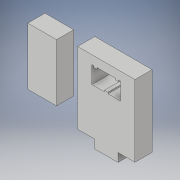
# Autodesk Inventor part: for_metabois
Saved by Autodesk Inventor 2019 (Build 230136000, 136)
## iProperties
Created: 2018-09-25
Part Number: for_metabois
Material: Générique
Document SubType Name: Modeling
Designer: Jérémy
Density: 1 g/cm^3
Appearance: Par défaut
Author: Jérémy
Autodesk Inventor part; units mm, degrees
ref_plane "YZ Plane" through (0, 0, 0) normal (1, 0, 0) x (0, 1, 0)
ref_plane "XZ Plane" through (0, 0, 0) normal (0, 1, 0) x (-1, 0, 0)
ref_plane "XY Plane" through (0, 0, 0) normal (0, 0, 1) x (1, 0, 0)
sketch "Esquisse1" plane through (0, 0, 0) normal (0, 0, 1) x (1, 0, 0)
  line L0 (-7.3739, 13.4012) -> (12.6261, 13.4012)
  line L1 (12.6261, 13.4012) -> (12.6261, -11.5988)
  line L2 (12.6261, -11.5988) -> (6.7261, -11.5988)
  line L3 (6.7261, -11.5988) -> (6.7261, -14.5988)
  line L4 (6.7261, -14.5988) -> (-1.4739, -14.5988)
  line L5 (-1.4739, -14.5988) -> (-1.4739, -11.5988)
  line L6 (-1.4739, -11.5988) -> (-7.3739, -11.5988)
  line L7 (-7.3739, -11.5988) -> (-7.3739, 13.4012)
  line L8 (-7.3739, 13.4012) -> (2.6261, 13.4012) construction
  line L9 (2.6261, 13.4012) -> (12.6261, 13.4012) construction
  line L10 (2.6261, 5.1758) -> (2.6261, -12.1236) construction
  line L11 (-1.4739, -14.5988) -> (2.6261, -14.5988) construction
  line L12 (2.6261, -14.5988) -> (6.7261, -14.5988) construction
  line L13 (-2.3739, 10.4012) -> (7.6261, 10.4012)
  line L14 (7.6261, 10.4012) -> (7.6261, 4.4012)
  line L15 (7.6261, 4.4012) -> (-2.3739, 4.4012)
  line L16 (-2.3739, 4.4012) -> (-2.3739, 10.4012)
  line L17 (-24.7357, 11.7717) -> (-14.7357, 11.7717)
  line L18 (-14.7357, 11.7717) -> (-14.7357, -8.2283)
  line L19 (-14.7357, -8.2283) -> (-24.7357, -8.2283)
  line L20 (-24.7357, -8.2283) -> (-24.7357, 11.7717)
  line L21 (-1.7739, 10.4012) -> (-1.7739, 9.9012)
  line L22 (-1.7739, 9.9012) -> (-0.5739, 9.9012)
  line L23 (-0.5739, 9.9012) -> (-0.5739, 10.4012)
  line L24 (5.8261, 10.4012) -> (5.8261, 9.9012)
  line L25 (5.8261, 9.9012) -> (7.0261, 9.9012)
  line L26 (7.0261, 9.9012) -> (7.0261, 10.4012)
  line L27 (2.0261, 4.4012) -> (2.0261, 4.9012)
  line L28 (2.0261, 4.9012) -> (3.2261, 4.9012)
  line L29 (3.2261, 4.9012) -> (3.2261, 4.4012)
  line L30 (-2.3739, 10.4012) -> (2.6261, 10.4012) construction
  line L31 (2.6261, 10.4012) -> (7.6261, 10.4012) construction
  point P0 (0, 0)
  point P1 (1, 1)
  dimension "d0" = 20
  dimension "d1" = 8.2
  dimension "d2" = 25
  dimension "d4" = 6
  dimension "d5" = 3
  dimension "d6" = 10
  dimension "d7" = 10
  dimension "d8" = 20
  dimension "d9" = 1.2
  dimension "d10" = 0.5
  dimension "d11" = 0.5
  dimension "d12" = 0.6
  dimension "d13" = 0.6
  dimension "d14" = 4.4
  dimension "d34" = 3
  constraints: 64 end point, 15 perpendicular, 13 point on line, 6 parallel, 5 equal length, 3 collinear, 3 horizontal, 3 midpoint
  measures "d0" distance of L0.start L0.end
  measures "d1" distance of L3.end L4.end
  measures "d2" distance of L0.end L1.end
  measures "d4" distance of L13.end L14.end
  measures "d5" vertical distance of L0.start L13.start
  measures "d6" distance of L14.end L15.end
  measures "d7" distance of L17.start L17.end
  measures "d8" distance of L19.end L17.start
  measures "d9" distance of L21.end L22.end
  measures "d10" distance of L28.end L29.end
  measures "d11" distance of L21.start L21.end
  measures "d12" horizontal distance of L13.start L21.end
  measures "d13" horizontal distance of L13.end L25.end
  measures "d14" horizontal distance of L15.end L27.end
  measures "d34" distance of L2.end L3.end
extrude "Extrusion1" add sketch "Esquisse1" along normal blind 6 contours L0 L1 L2 L3 L4 L5 L6 L7 | L13 L23 L22 L21 | L27 L28 L29 L15 | L13 L26 L25 L24 | L17 L18 L19 L20
equation "\"d0\" = L_modules"
equation "\"d1\" = L_metabois"
equation "\"d6\" = 0.5 * d0"
equation "\"d9\" = L_trou_int"
equation "\"d10\" = H_trou_int"
equation "\"d11\" = H_trou_int"
equation "\"d12\" = pos_trou_int_1"
equation "\"d13\" = pos_trou_int_1"
equation "\"d14\" = 0.5 * d6 - 0.5 * d9"
equation "\"d32\" = epaisseur_modules"
equation "\"epaisseur\" = 6"
equation "\"ecartement\" = 25"
equation "\"dvis\" = 3"
equation "\"largeur\" = 32"
equation "\"L_attache_carte\" = 15"
equation "\"marge_attache_carte\" = 5"
equation "\"L_cubi\" = 81.6"
equation "\"largeur_cubi\" = 81.6"
equation "\"L_moteur\" = 28.3"
equation "\"marge_trou\" = 2"
equation "\"taille_trou\" = 7"
equation "\"H_cubi\" = 81.6"
equation "\"epaisseur_wheel\" = 9"
equation "\"H_nez\" = 25"
equation "\"chanfrein\" = 0.5"
equation "\"H_trou_int\" = 0.5"
equation "\"L_trou_int\" = 1.2"
equation "\"pos_trou_int_1\" = 0.6"
equation "\"pos_trou_int_2\" = 2.9"
equation "\"epaisseur_metabois\" = 3"
equation "\"L_metabois\" = 8.2"
equation "\"epaisseur_modules\" = 6"
equation "\"L_modules\" = 20"
equation "\"d28\" = 8.2"
equation "\"d29\" = 1"
equation "\"d30\" = 0.4"
equation "\"d31\" = 0.5"
